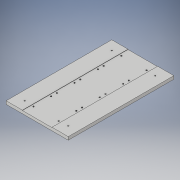
# Autodesk Inventor part: Assembly Plate
Saved by Autodesk Inventor 2019.4 (Build 234330000, 330)
## iProperties
Created: 2021-01-11
Part Number: Assembly Plate
Material: Generic
Document SubType Name: Modeling
Designer: caleb
Density: 1 g/cm^3
Appearance: Default
Author: caleb
Autodesk Inventor part; units mm, degrees
ref_plane "YZ Plane" through (0, 0, 0) normal (1, 0, 0) x (0, 1, 0)
ref_plane "XZ Plane" through (0, 0, 0) normal (0, 1, 0) x (-1, 0, 0)
ref_plane "XY Plane" through (0, 0, 0) normal (0, 0, 1) x (1, 0, 0)
sketch "Sketch1" plane through (0, 0, 0) normal (0, 1, 0) x (-1, 0, 0)
  line L0 (-63.5, 107.95) -> (63.5, 107.95)
  line L1 (63.5, 107.95) -> (63.5, -107.95)
  line L2 (63.5, -107.95) -> (-63.5, -107.95)
  line L3 (-63.5, -107.95) -> (-63.5, 107.95)
  line L4 (-63.5, 107.95) -> (63.5, -107.95) construction
  line L5 (63.5, 107.95) -> (-63.5, -107.95) construction
  point P0 (0, 0)
  dimension "d0" = 127
  dimension "d1" = 215.9
  constraints: 12 end point, 2 midpoint, 2 parallel, 1 horizontal, 1 perpendicular
  measures "d0" distance of L1.end L2.end
  measures "d1" distance of L0.end L1.end
extrude "Extrusion1" add sketch "Sketch1" along normal blind 6.35
sketch "Sketch5" plane through (0, 6.35, 0) normal (0, 1, 0) x (1, 0, 0)
  line L0 (-63.5, 107.95) -> (-63.5, -107.95) projected
  line L1 (-63.5, -107.95) -> (63.5, -107.95) projected
  point P0 (0, 0)
  point P1 (-44.45, -88.9)
  point P2 (-44.45, 88.9)
  point P3 (44.45, -88.9)
  point P4 (44.45, 88.9)
  dimension "d36" = 19.05
  dimension "d37" = 19.05
  dimension "d40" = 177.8
  dimension "d43" = 88.9
  constraints: 1 horizontal, 1 vertical, 3 other
  measures "d36" distance from line of L0 point (-44.45, -88.9)
  measures "d37" distance from line of L1 point (-44.45, -88.9)
  measures "d40" distance of point (-44.45, -88.9) point (-44.45, 88.9)
  measures "d43" distance of point (-44.45, -88.9) point (44.45, -88.9)
hole "Hole2" at (-44.45, 6.35, 88.9) at (-44.45, 6.35, -88.9) at (44.45, 6.35, 88.9) at (44.45, 6.35, -88.9) direction (0, -1, 0) diameter 2.4638 end through all
sketch "Sketch6" plane through (0, 6.35, 0) normal (0, 1, 0) x (1, 0, 0)
  line L0 (63.5, 107.95) -> (-63.5, 107.95) projected
  line L1 (30.25, -107.95) -> (-30.25, -107.95)
  line L2 (-30.25, -107.95) -> (-30.25, 107.95)
  line L3 (-30.25, 107.95) -> (30.25, 107.95)
  line L4 (30.25, 107.95) -> (30.25, -107.95)
  line L5 (30.25, -107.95) -> (-30.25, 107.95) construction
  line L6 (-30.25, -107.95) -> (30.25, 107.95) construction
  point P0 (0, 0)
  dimension "d53" = 60.5
  constraints: 12 end point, 2 midpoint, 2 parallel, 1 horizontal, 1 perpendicular, 1 point on line
  measures "d53" distance between parallel lines of L4 L2
extrude "Extrusion4" cut sketch "Sketch6" against normal blind 0.635
sketch "Sketch8" plane through (0, 5.715, 0) normal (0, 1, 0) x (1, 0, 0)
  circle A0 centre (-25.7556, -89.8398) radius 1.2
  line L0 (30.25, -107.95) -> (-30.25, -107.95) projected
  line L1 (-63.5, 107.95) -> (-63.5, -107.95) projected
  circle A1 centre (-25.7556, -53.7464) radius 1.2
  circle A2 centre (25.7556, -89.8398) radius 1.2
  circle A3 centre (25.7556, -53.7464) radius 1.2
  circle A4 centre (-25.7556, -41.9862) radius 1.2
  circle A5 centre (-25.7556, -5.8928) radius 1.2
  circle A6 centre (25.7556, -5.8928) radius 1.2
  circle A7 centre (25.7556, -41.9862) radius 1.2
  circle A8 centre (-25.7556, 5.8674) radius 1.2
  circle A9 centre (-25.7556, 41.9608) radius 1.2
  circle A10 centre (25.7556, 41.9608) radius 1.2
  circle A11 centre (25.7556, 5.8674) radius 1.2
  circle A12 centre (-25.7556, 53.721) radius 1.2
  circle A13 centre (-25.7556, 89.8144) radius 1.2
  circle A14 centre (25.7556, 89.8144) radius 1.2
  circle A15 centre (25.7556, 53.721) radius 1.2
  point P0 (0, 0)
  dimension "d56" = 2.4
  dimension "d57" = 18.1102
  dimension "d58" = 37.7444
  dimension "d59" = 36.0934
  dimension "d60" = 51.5112
  dimension "d63" = 47.8536
  constraints: 16 centre point, 3 equal radius, 2 horizontal alignment, 2 vertical alignment, 1 vertical, 24 other
  measures "d56" diameter of A0
  measures "d57" distance from line of L0 A0.centre
  measures "d58" distance from line of L1 A0.centre
  measures "d59" distance of A1.centre A0.centre
  measures "d60" distance of A2.centre A0.centre
  measures "d63" distance of A0.centre A4.centre
extrude "Extrusion5" add sketch "Sketch8" along normal blind 0.635
sketch "Sketch9" plane through (-25.7556, 6.35, 89.8398) normal (0, 1, 0) x (1, 0, 0)
  circle A0 centre (51.5112, 0) radius 1.2 projected
  circle A1 centre (51.5112, 36.0934) radius 1.2 projected
  circle A2 centre (51.5112, 47.8536) radius 1.2 projected
  circle A3 centre (0, 47.8536) radius 1.2 projected
  circle A4 centre (0, 36.0934) radius 1.2 projected
  circle A5 centre (51.5112, 83.947) radius 1.2 projected
  circle A6 centre (51.5112, 95.7072) radius 1.2 projected
  circle A7 centre (0, 95.7072) radius 1.2 projected
  circle A8 centre (0, 83.947) radius 1.2 projected
  circle A9 centre (51.5112, 131.8006) radius 1.2 projected
  circle A10 centre (0, 131.8006) radius 1.2 projected
  circle A11 centre (0, 143.5608) radius 1.2 projected
  circle A12 centre (51.5112, 143.5608) radius 1.2 projected
  circle A13 centre (51.5112, 179.6542) radius 1.2 projected
  circle A14 centre (0, 179.6542) radius 1.2 projected
  circle A15 centre (0, 0) radius 1.2 projected
  circle A16 centre (51.5112, 0) radius 1.2 projected
  circle A17 centre (51.5112, 83.947) radius 1.2 projected
  circle A18 centre (51.5112, 95.7072) radius 1.2 projected
  circle A19 centre (0, 95.7072) radius 1.2 projected
  circle A20 centre (0, 83.947) radius 1.2 projected
  circle A21 centre (51.5112, 131.8006) radius 1.2 projected
  circle A22 centre (51.5112, 143.5608) radius 1.2 projected
  circle A23 centre (51.5112, 179.6542) radius 1.2 projected
  point P0 (25.7556, 89.8398)
  constraints: 15 coincident
hole "Hole3" at (-25.7556, 6.35, 89.8398) at (25.7556, 6.35, 89.8398) at (25.7556, 6.35, 53.7464) at (25.7556, 6.35, 41.9862) at (-25.7556, 6.35, 41.9862) at (-25.7556, 6.35, 53.7464) at (25.7556, 6.35, 5.8928) at (25.7556, 6.35, -5.8674) at (-25.7556, 6.35, -5.8674) at (-25.7556, 6.35, 5.8928) at (25.7556, 6.35, -41.9608) at (25.7556, 6.35, -53.721) at (-25.7556, 6.35, -53.721) at (-25.7556, 6.35, -41.9608) at (-25.7556, 6.35, -89.8144) at (25.7556, 6.35, -89.8144) direction (0, -1, 0) diameter 1.5748 end through all
body "Solid1"
